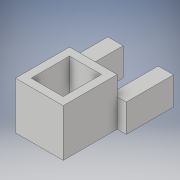
# Autodesk Inventor part: motorMount
Saved by Autodesk Inventor 2019 (Build 230136000, 136)
## iProperties
Created: 2023-04-04
Part Number: motorMount
Material: Generic
Document SubType Name: Modeling
Designer: Ella Moss
Density: 1 g/cm^3
Appearance: Default
Author: Ella Moss
Autodesk Inventor part; units mm, degrees
ref_plane "YZ Plane" through (0, 0, 0) normal (1, 0, 0) x (0, 1, 0)
ref_plane "XZ Plane" through (0, 0, 0) normal (0, 1, 0) x (-1, 0, 0)
ref_plane "XY Plane" through (0, 0, 0) normal (0, 0, 1) x (1, 0, 0)
sketch "Sketch1" plane through (0, 0, 0) normal (0, 1, 0) x (-1, 0, 0)
  line L0 (0, 0) -> (10.127, 0)
  line L1 (10.127, 0) -> (10.127, -12.127)
  line L2 (10.127, -12.127) -> (0, -12.127)
  line L3 (0, -12.127) -> (0, 0)
  line L4 (-2.5, 2.5) -> (12.627, 2.5)
  line L5 (12.627, 2.5) -> (12.627, -14.627)
  line L6 (12.627, -14.627) -> (-2.5, -14.627)
  line L7 (-2.5, -14.627) -> (-2.5, 2.5)
  dimension "d5" = 10.127
  dimension "d6" = 12.127
  dimension "d7" = 2.5
  dimension "d8" = 2.5
  dimension "d9" = 2.5
  dimension "d10" = 2.5
  constraints: 16 end point, 4 parallel, 2 horizontal, 2 perpendicular
  measures "d5" distance of L1.end L2.end
  measures "d6" distance of L0.end L1.end
  measures "d7" distance between parallel lines of L6 L2
  measures "d8" distance between parallel lines of L7 L3
  measures "d9" distance between parallel lines of L4 L0
  measures "d10" distance between parallel lines of L1 L5
extrude "Extrusion2" add sketch "Sketch1" along normal blind 15
sketch "Sketch3" plane through (2.5, 0, -14.627) normal (0, 0, -1) x (-1, 0, 0)
  line L0 (17.974, 0) -> (13.124, 0)
  line L1 (13.124, 0) -> (13.124, 8.85)
  line L2 (13.124, 8.85) -> (17.974, 8.85)
  line L3 (17.974, 8.85) -> (17.974, 0)
  line L4 (2.003, 0) -> (-2.847, 0)
  line L5 (-2.847, 0) -> (-2.847, 8.85)
  line L6 (-2.847, 8.85) -> (2.003, 8.85)
  line L7 (2.003, 8.85) -> (2.003, 0)
  line L8 (15.127, 0) -> (0, 0) projected
  line L9 (7.5635, 0) -> (7.5635, 15)
  line L10 (12.627, 15) -> (2.5, 15) projected
  dimension "d14" = 4.85
  dimension "d15" = 8.85
  dimension "d16" = 4.85
  dimension "d17" = 8.85
  dimension "d18" = 11.121
  constraints: 18 end point, 4 parallel, 2 horizontal, 2 midpoint, 2 perpendicular, 1 collinear, 1 point on line, 1 other
  measures "d14" distance of L0.start L0.end
  measures "d15" distance of L2.end L0.start
  measures "d16" distance of L4.start L4.end
  measures "d17" distance of L6.end L4.start
  measures "d18" distance between parallel lines of L7 L1
extrude "Extrusion3" add sketch "Sketch3" along normal blind 15
equation "\"d8\" = d7"
equation "\"d9\" = d7"
equation "\"d10\" = d7"
body "Solid2"
